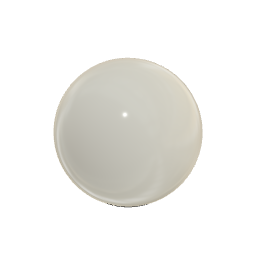
EXAMPLE_Butyric_acid_v4 (Autodesk Fusion 360 archive; units mm, degrees)
design "Hidrogenia"
Autodesk Fusion 360 part; units mm, degrees
sketch "Sketch1" plane through (0, 0, 0) normal (0, 1, 0) x (1, 0, 0)
  circle A0 centre (0, 0) radius 9.7059
  line L0 (0, -9.7059) -> (0, 9.7059)
  dimension "d1" = 19.4118
  constraint coincident A0.centre origin
  constraint coincident A0 L0.start
  constraint coincident A0 L0.end
  constraint vertical L0
  measures "d1" diameter of A0
revolve "Revolve1" add sketch "Sketch1" angle 360 about axis through (0, 0, 9.7059) along (0, 0, -1) contours A0 L0 picked at (2.6606, -2.8528)
sketch "Sketch2" plane through (0, 0, 0) normal (0, 1, 0) x (1, 0, 0)
  circle A0 centre (0, 0) radius 9.7059 construction
  line L0 (0, -9.7059) -> (0, 9.7059)
  line L1 (0, 9.7059) -> (5, 9.7059)
  line L2 (5, 9.7059) -> (5, 8.3189)
  line L3 (5, 8.3189) -> (2.5, 8.3189)
  line L4 (2.5, 8.3189) -> (2.5, 5.3189)
  line L5 (2.5, 5.3189) -> (0, 5.3189)
  dimension "d5" = 2.5
  dimension "d9" = 5
  dimension "d10" = 3
  constraint coincident A0 L0.start
  constraint coincident A0 L0.end
  constraint vertical L0
  constraint coincident A0.centre L0
  constraint tangent A0 L1
  constraint perpendicular L1 L2
  constraint perpendicular L2 L3
  constraint perpendicular L3 L4
  constraint coincident L0 L5.end
  constraint perpendicular L0 L5
  constraint coincident A0 L2.end
  measures "d5" distance of L0 L4
  measures "d9" distance of L0.end L1.end
  measures "d10" distance of L3.end L4.end
revolve "Revolve2" cut sketch "Sketch2" angle 360 about axis through (0, 0, 9.7059) along (0, 0, -1)
fillet "Fillet1" radius 0.4 1 edges at (-2.3308, -0.904, -8.3189)
equation "d1 = atomsize"
equation "atomsize = ( 110 / ( 170 / 30 ) ) * 1 mm"
equation "a_size = ( ( atomsize * 2 ) / ( ( 6 ) ^ ( 1 / 2 ) ) )"
